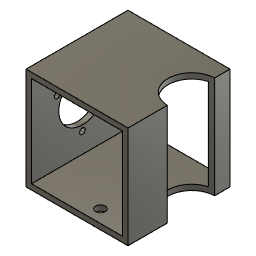
Roller+em+ferro+(Cubo) (Autodesk Fusion 360 design; units mm, degrees)
Autodesk Fusion 360 part; units mm, degrees
sketch "Esboço1" plane through (0, 0, 0) normal (0, 1, 0) x (1, 0, 0)
  line L0 (0, 0) -> (56, 0)
  line L1 (56, -56) -> (0, -56)
  line L2 (0, -56) -> (0, 0)
  line L3 (0, -28) -> (45.1892, -28)
  arc A0 (56, -8.4245) -> (56, -34.4121) centre (56.4, -21.4183) ccw
  line L4 (56, 0) -> (56, -8.4245)
  line L5 (56, -34.4121) -> (56, -56)
  circle A1 centre (24.93, -7) radius 2.65
  circle A2 centre (33.9, -49) radius 2.65
  dimension "d1" = 56
  dimension "d2" = 56
  dimension "d3" = 26
  dimension "d5" = 5.3
  dimension "d6" = 24.93
  dimension "d7" = 21
  dimension "d8" = 5.3
  dimension "d9" = 21
  dimension "d10" = 33.9
  dimension "d47" = 56.4
  constraint horizontal L0
  constraint vertical L4
  constraint horizontal L1
  constraint vertical L2
  constraint coincident L0.start L2.end
  constraint midpoint L2 L3.start
  constraint coincident A0.end L4
  constraint collinear L4 L5
  constraint coincident A0 L3.end
  measures "d1" distance of L0.start L0.end
  measures "d2" distance of L0.start L1.end
  measures "d3" diameter of A0
  measures "d5" diameter of A1
  measures "d6" distance of L2 A1.centre
  measures "d7" distance of L3 A1.centre
  measures "d8" diameter of A2
  measures "d9" distance of L3 A2.centre
  measures "d10" distance of L2 A2.centre
  measures "d47" distance of L2 A0.centre
extrude "Extrusão1" add sketch "Esboço1" along normal blind 3
sketch "Esboço2" plane through (0, 3, 0) normal (0, 1, 0) x (-1, 0, 0)
  circle A0 centre (-24.93, 7) radius 2.65
  circle A1 centre (-33.9, 49) radius 2.65
  arc A2 (-56, 8.4245) -> (-56, 34.4121) centre (-56.4, 21.4183) ccw
  line L0 (-56, 8.4245) -> (-56, 0)
  line L1 (-56, 0) -> (0, 0)
  line L2 (0, 0) -> (0, 56)
  line L3 (0, 56) -> (-56, 56)
  line L4 (-56, 56) -> (-56, 34.4121)
  line L5 (0, 0) -> (-3, 0)
  line L6 (-3, 0) -> (-3, 56)
  line L7 (-3, 56) -> (0, 56)
  line L8 (0, 56) -> (0, 0)
  constraint horizontal L5
  constraint vertical L6
  constraint horizontal L7
  constraint vertical L8
  constraint coincident L3 L6.end
  constraint coincident L1.end L2.start
extrude "Extrusão2" add sketch "Esboço2" along normal blind 53 contours L1 L2 L3 L5 L6 L7 L8
sketch "Esboço3" plane through (0, 0, 0) normal (-1, 0, 0) x (0, 0, 1)
  line L0 (0, 0) -> (56, 0)
  line L1 (56, 0) -> (56, 56)
  line L2 (56, 56) -> (0, 56)
  line L3 (0, 56) -> (0, 0)
  circle A0 centre (28, 30) radius 13
  circle A1 centre (28, 14) radius 1.6
  circle A2 centre (14.1436, 38) radius 1.6
  circle A3 centre (41.8564, 38) radius 1.6
  dimension "d15" = 26
  dimension "d16" = 30
  dimension "d19" = 3.2
  dimension "d20" = 16
  dimension "d21" = 8
  dimension "d22" = 13.8564
  measures "d15" diameter of A0
  measures "d16" distance of L0 A0.centre
  measures "d19" diameter of A1
  measures "d20" distance of A0.centre A1.centre
  measures "d21" vertical distance of A0.centre A3.centre
  measures "d22" horizontal distance of A0.centre A3.centre
extrude "Extrusão3" cut sketch "Esboço3" against normal blind 6.5 contours A0 | A1 | A2 | A3
sketch "Esboço6" plane through (3, 0, 0) normal (1, 0, 0) x (0, 0, -1)
  circle A0 centre (-41.8564, 38) radius 1.6
  circle A1 centre (-28, 14) radius 1.6
  circle A2 centre (-14.1436, 38) radius 1.6
  circle A3 centre (-28, 30) radius 13
  line L0 (-56, 3) -> (0, 3)
  line L1 (0, 3) -> (0, 56)
  line L2 (0, 56) -> (-56, 56)
  line L3 (-56, 56) -> (-56, 3)
  line L4 (-56, 56) -> (0, 56)
  line L5 (0, 56) -> (0, 53)
  line L6 (0, 53) -> (-56, 53)
  line L7 (-56, 53) -> (-56, 56)
  dimension "d48" = 3
  constraint horizontal L4
  constraint vertical L5
  constraint horizontal L6
  constraint vertical L7
  constraint coincident L2.end L3.start
  measures "d48" distance of L2.end L6.end
extrude "Extrusão6" add sketch "Esboço6" along normal blind 53 contours L1 L2 L3 L4 L5 L6 L7
sketch "Esboço7" plane through (0, 53, 0) normal (0, -1, 0) x (1, 0, 0)
  line L0 (3, 56) -> (3, 0)
  line L1 (3, 0) -> (56, 0)
  line L2 (56, 0) -> (56, 56)
  line L3 (56, 56) -> (3, 56)
  line L4 (56, 0) -> (53, 0)
  line L5 (53, 0) -> (53, 56)
  line L6 (53, 56) -> (56, 56)
  line L7 (56, 56) -> (56, 0)
  dimension "d51" = 3
  constraint horizontal L4
  constraint vertical L5
  constraint horizontal L6
  constraint vertical L7
  constraint coincident L1.end L2.start
  measures "d51" distance of L1.end L4.end
extrude "Extrusão7" add sketch "Esboço7" along normal blind 50 contours L1 L2 L3 L4 L5 L6 L7
sketch "Esboço8" plane through (0, 0, 0) normal (0, -1, 0) x (1, 0, 0)
  circle A0 centre (33.9, 49) radius 2.65
  circle A1 centre (24.93, 7) radius 2.65
  arc A2 (56, 34.4121) -> (56, 8.4245) centre (56.4, 21.4183) ccw
  line L0 (56, 34.4121) -> (56, 56)
  line L1 (56, 56) -> (0, 56)
  line L2 (0, 56) -> (0, 0)
  line L3 (0, 0) -> (56, 0)
  line L4 (56, 0) -> (56, 8.4245)
  circle A3 centre (56.4, 21.4183) radius 13
  constraint concentric A2 A3
extrude "Extrusão8" cut sketch "Esboço8" against normal blind 69 contours A2 A3
